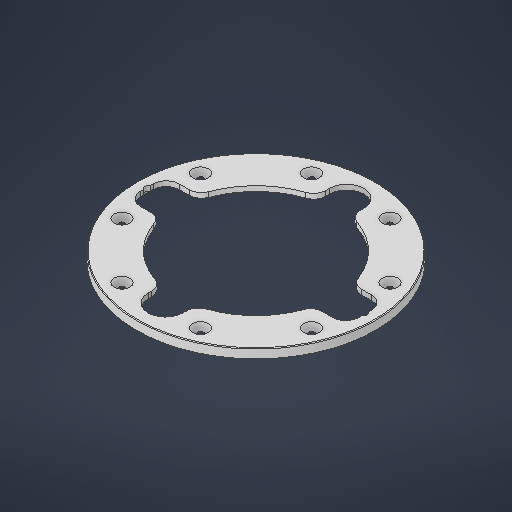
# Autodesk Inventor part: Clamp Ring
Saved by Autodesk Inventor 2025 (Build 290162000, 162)
## iProperties
Created: 2024-08-23
Part Number: Clamp Ring
Material: Generic
Document SubType Name: Modeling
Designer: mayhe
Density: 1 g/cm^3
Appearance: Default
Author: mayhe
Autodesk Inventor part; units mm, degrees
ref_plane "YZ Plane" through (0, 0, 0) normal (1, 0, 0) x (0, 1, 0)
ref_plane "XZ Plane" through (0, 0, 0) normal (0, 1, 0) x (-1, 0, 0)
ref_plane "XY Plane" through (0, 0, 0) normal (0, 0, 1) x (1, 0, 0)
sketch "Sketch1" plane through (0, 0, 0) normal (0, 1, 0) x (-1, 0, 0)
  circle A0 centre (0, 0) radius 84.5
  circle A1 centre (0, 0) radius 80.5
  constraints: 2 centre point, 1 coincident
extrude "Extrusion1" add sketch "Sketch1" along normal blind 6.5
extrude "Extrusion2" add sketch "Sketch1" along normal blind 3.5 contours A1
sketch "Sketch2" plane through (0, 0, 0) normal (0, -1, 0) x (1, 0, 0)
  circle A0 centre (0, 0) radius 72.5
  circle A1 centre (0, 72.5) radius 1
  line L0 (0, 0) -> (-102.6766, 42.53)
  line L1 (0, 0) -> (-104.775, 0)
  circle A2 centre (-66.9813, 27.7445) radius 2.5
  circle A3 centre (-66.9813, -27.7445) radius 2.5
  circle A4 centre (-27.7445, -66.9813) radius 2.5
  circle A5 centre (27.7445, -66.9813) radius 2.5
  circle A6 centre (66.9813, -27.7445) radius 2.5
  circle A7 centre (66.9813, 27.7445) radius 2.5
  circle A8 centre (27.7445, 66.9813) radius 2.5
  circle A9 centre (-27.7445, 66.9813) radius 2.5
  point P0 (36.25, -62.7868)
  point P1 (62.7868, -36.25)
  point P2 (72.5, 0)
  point P3 (62.7868, 36.25)
  point P4 (36.25, 62.7868)
  point P5 (-36.25, 62.7868)
  point P6 (-62.7868, 36.25)
  point P7 (-72.5, 0)
  point P8 (-62.7868, -36.25)
  point P9 (-36.25, -62.7868)
  dimension "d14" = 145
  dimension "d15" = 2
  dimension "d87" = 22.5
  dimension "d88" = 5
  dimension "d91" = 360
  constraints: 10 centre point, 4 end point, 2 point on circle, 1 coincident, 1 horizontal, 1 point on line, 17 other
  measures "d14" diameter of A0
  measures "d15" diameter of A1
  measures "d87" angle of L0 L1
  measures "d88" diameter of A2
hole "Hole1" at (-72.5, 0, 0) at (72.5, 0, 0) direction (0, 1, 0) diameter 3.5 depth 8.8
chamfer "Chamfer2" distance 0.5 angle 45 1 edges at (84.5, 0, 0)
hole "Hole2" at (27.7445, 0, -66.9813) at (-27.7445, 0, -66.9813) at (-66.9813, 0, -27.7445) at (-66.9813, 0, 27.7445) at (-27.7445, 0, 66.9813) at (27.7445, 0, 66.9813) at (66.9813, 0, 27.7445) at (66.9813, 0, -27.7445) direction (0, 1, 0) diameter 4.134 depth 14.2 countersink diameter 11.2 countersink angle 90 thread size "M5x0.8" class "6H" standard "ISO Metric profile"
sketch "Sketch4" plane through (0, 0, 0) normal (0, -1, 0) x (1, 0, 0)
  line L0 (-76, -4.5) -> (-76, 4.5)
  arc A0 (-76, -4.5) -> (-68, -12.5) centre (-68, -4.5) ccw
  line L1 (-68, -4.5) -> (-68, -12.5) construction
  line L2 (-68, -4.5) -> (-76, -4.5) construction
  arc A1 (-68, 12.5) -> (-76, 4.5) centre (-68, 4.5) ccw
  line L3 (-68, -12.5) -> (-61.0376, -12.5)
  line L4 (-68, 12.5) -> (-60.9816, 12.5)
  arc A2 (-60.9816, 12.5) -> (-51.5998, 19.0385) centre (-60.9816, 22.5) ccw
  arc A3 (-52.0335, -17.819) -> (-61.0376, -12.5) centre (-60.2612, -21.4665) ccw
  line L5 (-10.9, -64.1) -> (-10.9, -61.5483)
  arc A4 (-10.9, -61.5483) -> (-17.6846, -52.0793) centre (-20.9, -61.5483) ccw
  arc A5 (17.6846, -52.0793) -> (10.9, -61.5483) centre (20.9, -61.5483) ccw
  line L6 (10.9, -64.1) -> (10.9, -61.5483)
  arc A6 (-10.9, -64.1) -> (10.9, -64.1) centre (0, -64.1) ccw
  circle A7 centre (0, 0) radius 84 projected
  line L7 (0, 0) -> (0, 55)
  line L8 (0, 0) -> (55, 0)
  arc A8 (-17.6846, 52.0793) -> (-10.9, 61.5483) centre (-20.9, 61.5483) ccw
  line L9 (-10.9, 64.1) -> (-10.9, 61.5483)
  line L10 (10.9, 64.1) -> (10.9, 61.5483)
  arc A9 (10.9, 61.5483) -> (17.6846, 52.0793) centre (20.9, 61.5483) ccw
  arc A10 (10.9, 64.1) -> (-10.9, 64.1) centre (0, 64.1) ccw
  arc A11 (61.0376, -12.5) -> (52.0335, -17.819) centre (60.2612, -21.4665) ccw
  line L11 (76, -4.5) -> (76, 4.5)
  arc A12 (51.5998, 19.0385) -> (60.9816, 12.5) centre (60.9816, 22.5) ccw
  line L12 (68, -4.5) -> (68, -12.5) construction
  line L13 (68, -12.5) -> (61.0376, -12.5)
  line L14 (68, 12.5) -> (60.9816, 12.5)
  arc A13 (68, -12.5) -> (76, -4.5) centre (68, -4.5) ccw
  line L15 (68, -4.5) -> (76, -4.5) construction
  arc A14 (76, 4.5) -> (68, 12.5) centre (68, 4.5) ccw
  arc A15 (-17.6846, 52.0793) -> (-51.5998, 19.0385) centre (0, 0) ccw
  arc A16 (51.5998, 19.0385) -> (17.6846, 52.0793) centre (0, 0) ccw
  arc A17 (-52.0335, -17.819) -> (-17.6846, -52.0793) centre (0, 0) ccw
  arc A18 (17.6846, -52.0793) -> (52.0335, -17.819) centre (0, 0) ccw
  arc A19 (12.15, 61.5483) -> (18.0865, 53.2629) centre (20.9, 61.5483) ccw
  line L16 (12.15, 61.5483) -> (12.15, 64.1)
  arc A20 (12.15, 64.1) -> (-12.15, 64.1) centre (0, 64.1) ccw
  line L17 (-12.15, 64.1) -> (-12.15, 61.5483)
  arc A21 (-18.0865, 53.2629) -> (-12.15, 61.5483) centre (-20.9, 61.5483) ccw
  arc A22 (-18.0865, 53.2629) -> (-52.7725, 19.4712) centre (0, 0) ccw
  arc A23 (-60.9816, 13.75) -> (-52.7725, 19.4712) centre (-60.9816, 22.5) ccw
  line L18 (-60.9816, 13.75) -> (-68, 13.75)
  arc A24 (-68, 13.75) -> (-77.25, 4.5) centre (-68, 4.5) ccw
  line L19 (-77.25, 4.5) -> (-77.25, -4.5)
  arc A25 (-77.25, -4.5) -> (-68, -13.75) centre (-68, -4.5) ccw
  line L20 (-68, -13.75) -> (-60.9816, -13.75)
  arc A26 (-52.7725, -19.4712) -> (-60.9816, -13.75) centre (-60.2612, -21.4665) ccw
  arc A27 (-52.7725, -19.4712) -> (-18.0865, -53.2629) centre (0, 0) ccw
  arc A28 (-12.15, -61.5483) -> (-18.0865, -53.2629) centre (-20.9, -61.5483) ccw
  line L21 (-12.15, -61.5483) -> (-12.15, -64.1)
  arc A29 (-12.15, -64.1) -> (12.15, -64.1) centre (0, -64.1) ccw
  line L22 (12.15, -64.1) -> (12.15, -61.5483)
  arc A30 (18.0865, -53.2629) -> (12.15, -61.5483) centre (20.9, -61.5483) ccw
  arc A31 (18.0865, -53.2629) -> (52.7725, -19.4712) centre (0, 0) ccw
  arc A32 (60.9816, -13.75) -> (52.7725, -19.4712) centre (60.2612, -21.4665) ccw
  line L23 (60.9816, -13.75) -> (68, -13.75)
  arc A33 (68, -13.75) -> (77.25, -4.5) centre (68, -4.5) ccw
  line L24 (77.25, -4.5) -> (77.25, 4.5)
  arc A34 (77.25, 4.5) -> (68, 13.75) centre (68, 4.5) ccw
  line L25 (68, 13.75) -> (60.9816, 13.75)
  arc A35 (52.7725, 19.4712) -> (60.9816, 13.75) centre (60.9816, 22.5) ccw
  arc A36 (52.7725, 19.4712) -> (18.0865, 53.2629) centre (0, 0) ccw
  dimension "d77" = 90
  dimension "d78" = 8
  dimension "d79" = 25
  dimension "d80" = 76
  dimension "d81" = 10
  dimension "d82" = 64.1
  dimension "d83" = 10
  dimension "d84" = 10.9
  dimension "d85" = 1.25
  dimension "d86" = 8
  constraints: 72 point on circle, 52 end point, 36 centre point, 21 symmetric about line, 5 tangent, 3 vertical, 2 horizontal, 1 coincident, 1 perpendicular, 34 other
  measures "d77" angle of L2 L1
  measures "d78" radius of A0
  measures "d79" distance of L4.start L1.end
  measures "d80" distance from line of point (0, 0) L0
  measures "d81" radius of A2
  measures "d82" distance of point (0, 0) A6.centre
  measures "d83" radius of A4
  measures "d84" radius of A6
  measures "d85" radial gap between concentric circles of A16 A36
  measures "d86" radius of A1
extrude "Extrusion4" cut sketch "Sketch4" against normal blind 10 contours L0 A1 L4 A2 A15 A8 L9 A10 L10 A9 A16 A12 L14 A14 L11 A13 L13 A11 A18 A5 L6 A6 L5 A4 A17 A3 L3 A0 | A19 A36 A35 L25 A34 L24 A33 L23 A32 A31 A30 L22 A29 L21 A28 A27 A26 L20 A25 L19 A24 L18 A23 A22 A21 L17 A20 L16
sketch "Sketch5" plane through (0, 0, 0) normal (0, -1, 0) x (1, 0, 0)
  circle A0 centre (0, 0) radius 76
  circle A1 centre (-76, 0) radius 2.5
  circle A2 centre (76, 0) radius 2.5
  dimension "d93" = 5
  dimension "d94" = 5
  dimension "d102" = 152
  constraints: 3 centre point, 2 point on circle, 1 coincident
  measures "d93" diameter of A1
  measures "d94" diameter of A2
  measures "d102" diameter of A0
hole "Hole4" at (-76, 0, 0) at (76, 0, 0) direction (0, 1, 0) diameter 5.5 depth 14.2
body "Solid1"
